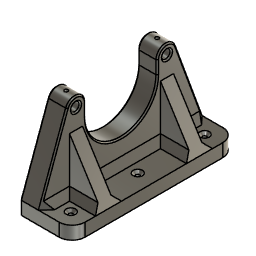
Slider Rod Bracket v4 (Autodesk Fusion 360 design; units mm, degrees)
Autodesk Fusion 360 part; units mm, degrees
sketch "Sketch1" plane through (0, 0, 0) normal (1, 0, 0) x (0, 1, 0)
  circle A0 centre (0, 0) radius 3.275
  circle A1 centre (70, 0) radius 3.275
  circle A2 centre (0, 0) radius 7.5
  circle A3 centre (70, 0) radius 7.5
  line L0 (70, 0) -> (70, -65) construction
  line L1 (7.5, 0) -> (7.5, -10)
  line L2 (70, -65) -> (-73.8132, -65) construction
  line L3 (62.5, 0) -> (62.5, -10)
  line L4 (-27.9997, -55) -> (97.9997, -55)
  line L5 (-7.0477, 2.5652) -> (-27.9997, -55)
  line L6 (0, 0) -> (70, 0) construction
  line L7 (35, 0) -> (35, -33.7499) construction
  line L8 (77.0477, 2.5652) -> (97.9997, -55)
  circle A4 centre (35, -10) radius 27.5
  line L9 (-27.9997, -55) -> (-27.9997, -65)
  line L10 (97.9997, -55) -> (97.9997, -65)
  line L11 (97.9997, -65) -> (-27.9997, -65)
  dimension "d1" = 6.55
  dimension "d2" = 6.55
  dimension "d3" = 70
  dimension "d4" = 15
  dimension "d5" = 15
  dimension "d6" = 65
  dimension "d7" = 10
  dimension "d8" = 10
  dimension "d9" = 10
  dimension "d10" = 70
  dimension "d11" = 10
  constraint coincident A0.centre A2.centre
  constraint horizontal A0.centre A1.centre
  constraint concentric A0 A2
  constraint concentric A1 A3
  constraint coincident A1.centre A3.centre
  constraint vertical L0
  constraint coincident A2 L1.start
  constraint tangent A2 L1
  constraint vertical L1
  constraint horizontal L2
  constraint coincident A3 L3.start
  constraint vertical L3
  constraint tangent A3 L3
  constraint horizontal L4
  constraint coincident A2 L5.start
  constraint coincident L4 L5.end
  constraint tangent A2 L5
  constraint coincident L4.start L5.end
  constraint midpoint L6 L7.start
  constraint perpendicular L6 L7
  constraint symmetric L5.start L7 L8.start
  constraint symmetric L4.start L7 L4.end
  constraint coincident L4.end L8.end
  constraint tangent L3 A4
  constraint tangent L1 A4
  constraint horizontal L3.end A4.centre
  constraint coincident L2 L9.end
  constraint perpendicular L2 L9
  constraint perpendicular L4 L10
  measures "d1" diameter of A0
  measures "d2" diameter of A1
  measures "d3" distance of A0.centre A1.centre
  measures "d4" diameter of A2
  measures "d5" diameter of A3
  measures "d6" distance of A1.centre L0.end
  measures "d7" distance of L1.start L1.end
  measures "d8" distance of L3.start L3.end
  measures "d9" distance of L2 L4
  measures "d10" angle of L4 L5
  measures "d11" distance of L4.end L10.end
extrude "Extrude1" add sketch "Sketch1" against normal blind 15 contours A2 | A2 A3 L1 L3 L4 L5 L8 A4 | L4 L9 L10 L11 | A3
extrude "Extrude2" add sketch "Sketch1" along normal blind 25 contours L4 L9 L10 L11
ref_plane "WorkPlane1" through (0, 35, -16.8749) normal (0, 1, 0) x (0, 0, -1)
ref_plane "WorkPlane2" through (0, 0, -16.8749) normal (0, 1, 0) x (0, 0, -1)
sketch "Sketch2" plane through (0, 0, 0) normal (0, 1, 0) x (1, 0, 0)
  line L0 (0, -2.5652) -> (0, 55)
  line L1 (0, 55) -> (25, 55)
  line L2 (0, 15) -> (25, 55)
  point P0 (0, 55)
  dimension "d18" = 25
  dimension "d19" = 40
  constraint coincident L0 L2.start
  constraint coincident L1 L2.end
  measures "d18" distance of P0 L1.end
  measures "d19" distance of L2.start P0
extrude "Extrude3" add sketch "Sketch2" along normal mid plane 10
mirror "Mirror1" about plane through (0, 35, -16.8749) normal (0, 1, 0) of "Extrude3"
sketch "Sketch3" plane through (0, 0, -55) normal (0, 0, 1) x (-1, 0, 0)
  line L0 (-25, -65) -> (0, -65)
  line L1 (0, -65) -> (0, -5)
  line L2 (0, -5) -> (-25, -5)
  line L3 (-25, -5) -> (-25, -65)
  line L4 (-12.5, -65) -> (-12.5, -5) construction
  line L5 (-25, -35) -> (0, -35) construction
  circle A0 centre (-12.5, -35) radius 1.6
  line L6 (-25, -97.9997) -> (-25, -75)
  line L7 (-25, 5) -> (-25, 27.9997)
  line L8 (-25, -86.4998) -> (-12.5, -86.4998) construction
  circle A1 centre (-12.5, -86.4998) radius 1.6
  circle A2 centre (-12.5, 16.4998) radius 1.6
  dimension "d24" = 3.2
  dimension "d25" = 3.2
  constraint midpoint L0 L4.start
  constraint midpoint L2 L4.end
  constraint midpoint L3 L5.start
  constraint midpoint L1 L5.end
  constraint midpoint L5 A0.centre
  constraint midpoint L6 L8.start
  constraint perpendicular L4 L8
  constraint vertical L4.start L8.end
  constraint coincident L8.end A1.centre
  constraint symmetric L5 A1 A2
  measures "d24" diameter of A0
  measures "d25" diameter of A1
extrude "Extrude4" cut sketch "Sketch3" against normal blind 40 contours A0 | A1 | A2
chamfer "Chamfer1" distance 2 angle 45 3 edges at (13.9917, -17.0784, -55) (13.9917, 34.4214, -55) (13.9917, 85.9213, -55)
fillet "Fillet1" radius 10 2 edges at (25, -27.9997, -60) (25, 97.9997, -60)
chamfer "Chamfer2" distance 1 angle 45 9 edges at (0, -3.0534, 1.1843) (0, 66.9466, 1.1843) (0, 68.6976, 7.3861) (0, 62.5, -5) (0, 35, -37.5) (0, 7.5, -5) (0, 1.3024, 7.3861) (0, -17.5237, -26.2174) (0, 87.5237, -26.2174) 1 faces at (-15, 34.315, -55.8077)
chamfer "Chamfer3" distance 5 angle 45 7 edges at (0, -15.9678, -55) (12.5, -5, -55) (0, 35, -55) (12.5, 65, -55) (0, 85.9678, -55) (12.5, 75, -55) (12.5, 5, -55)
ref_plane "WorkPlane3" through (-7.5256, 70, 7.5) normal (0, 0, 1) x (0, -1, 0)
sketch "Sketch4" plane through (0, 0, 7.5) normal (0, 0, 1) x (1, 0, 0)
  line L0 (-1, 73.275) -> (-1, 66.725)
  line L1 (-14, 66.725) -> (-14, 73.275)
  line L2 (-1, 70) -> (-14, 70) construction
  circle A0 centre (-7.5, 70) radius 1.35
  dimension "d34" = 2.7
  constraint midpoint L0 L2.start
  constraint midpoint L1 L2.end
  constraint midpoint L2 A0.centre
  measures "d34" diameter of A0
extrude "Extrude5" cut sketch "Sketch4" against normal blind 7
mirror "Mirror2" about plane through (0, 35, -16.8749) normal (0, 1, 0) of "Extrude5"
